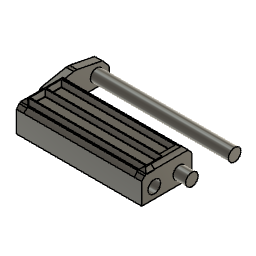
oruga v3 (Autodesk Fusion 360 design; units mm, degrees)
Autodesk Fusion 360 part; units mm, degrees
sketch "Sketch1" plane through (0, 0, 0) normal (0, 0, 1) x (1, 0, 0)
  line L0 (0, 0) -> (50, 0)
  line L1 (50, 0) -> (50, 20)
  line L2 (50, 20) -> (0, 20)
  line L3 (0, 20) -> (0, 0)
  constraint horizontal L0
  constraint vertical L1
  constraint horizontal L2
  constraint vertical L3
  constraint coincident L0.start L3.end
extrude "Extrude1" add sketch "Sketch1" along normal blind 10 contours L0 L1 L2 L3 picked at (16.666667, 13.333333) makes body 1
sketch "Sketch2" plane through (0, 0, 10) normal (0, 0, 1) x (-1, 0, 0)
  line L0 (0, -20) -> (0, 0)
  line L1 (0, 0) -> (-50, 0)
  line L2 (-50, 0) -> (-50, -20)
  line L3 (-50, -20) -> (0, -20)
  line L4 (0, -10) -> (-50, -10)
  line L5 (0, -20) -> (-50, -20)
  line L6 (-50, -20) -> (-50, 0)
  line L7 (-50, 0) -> (0, 0)
  line L8 (0, 0) -> (0, -20)
  line L9 (0, -10) -> (0, -11.5)
  line L10 (0, -10) -> (0, -8.5)
  line L11 (-25, -10) -> (-23.5, -10)
  line L12 (-25, -10) -> (-26.5, -10)
  line L13 (-23.5, -10) -> (-23.5, -20)
  line L14 (-23.5, -10) -> (-23.5, 0)
  line L15 (-26.5, -10) -> (-26.5, 0)
  line L16 (-26.5, -10) -> (-26.5, -20)
  line L17 (0, -20) -> (0, -15)
  line L18 (0, -15) -> (-50, -15)
  line L19 (0, 0) -> (0, -5)
  line L20 (-50, -5) -> (0, -5)
  line L21 (0, -5) -> (0, -2)
  line L22 (0, -2) -> (-1, -2)
  line L23 (-1, -2) -> (-50.000001, -2)
  line L24 (-50, -5) -> (-50.000001, -2)
  line L25 (0, -15) -> (0, -17.5)
  line L26 (0, -15) -> (0, -18)
  line L27 (0, -18) -> (-50, -18)
  line L28 (-50, -18) -> (-50, -15)
  line L29 (0, -10) -> (0, -11.5)
  line L30 (0, -10) -> (0, -8.5)
  line L31 (0, -11.5) -> (-50, -11.5)
  line L32 (0, -8.5) -> (-50, -8.5)
  line L33 (0, -20) -> (-2.713572, -20)
  line L34 (0, -20) -> (0, 0)
  line L35 (0, 0) -> (-2.713572, 0)
  line L36 (0, 0) -> (-2.713572, 0)
  line L37 (-50, -20) -> (-49.000001, -20)
  line L38 (-50, -20) -> (-48.000001, -20)
  line L39 (-50, 0) -> (-48.000001, 0)
  line L40 (0, -20) -> (-3, -20)
  line L41 (-3, -20) -> (-3, 0)
  line L42 (0, 0) -> (-3, 0)
  line L43 (-50, -20) -> (-47.000001, -20)
  line L44 (-47.000001, 0) -> (-47.000001, -20)
  line L45 (-47.000001, 0) -> (-50, 0)
  dimension "d5" = 1.5
  dimension "d6" = 1.5
  dimension "d7" = 3
  dimension "d8" = 3
  dimension "d9" = 1.5
  dimension "d10" = 3
  dimension "d13" = 1.5
  dimension "d22" = 2
  dimension "d23" = 2
  constraint midpoint L0 L4.start
  constraint midpoint L2 L4.end
  constraint horizontal L5
  constraint vertical L6
  constraint horizontal L7
  constraint vertical L8
  constraint coincident L1.end L2.start
  constraint coincident L0.start L3.end
  constraint perpendicular L4 L9
  constraint vertical L10
  constraint midpoint L4 L11.start
  constraint horizontal L11
  constraint horizontal L12
  constraint coincident L5 L13.end
  constraint perpendicular L5 L13
  constraint coincident L1 L14.end
  constraint perpendicular L1 L14
  constraint coincident L7 L15.end
  constraint perpendicular L7 L15
  constraint coincident L5 L16.end
  constraint perpendicular L5 L16
  constraint coincident L8 L17.end
  constraint coincident L6 L18.end
  constraint perpendicular L6 L18
  constraint coincident L0.end L1.start
  constraint coincident L8 L19.end
  constraint coincident L6 L20.start
  constraint perpendicular L0 L20
  constraint perpendicular L20 L21
  constraint perpendicular L8 L22
  constraint perpendicular L8 L23
  constraint perpendicular L23 L24
  constraint midpoint L17 L25.end
  constraint perpendicular L18 L26
  constraint coincident L6 L27.end
  constraint perpendicular L6 L27
  constraint perpendicular L4 L29
  constraint coincident L0 L10.end
  constraint coincident L6 L31.end
  constraint perpendicular L6 L31
  constraint coincident L6 L32.end
  constraint perpendicular L6 L32
  constraint perpendicular L17 L33
  constraint perpendicular L19 L35
  constraint coincident L2.end L3.start
  constraint perpendicular L2 L37
  constraint perpendicular L2 L38
  constraint perpendicular L8 L40
  constraint coincident L1 L41.end
  constraint perpendicular L1 L41
  constraint parallel L3 L43
  constraint perpendicular L5 L44
  measures "d5" distance of L11.start L11.end
  measures "d6" distance of L11.start L12.end
  measures "d7" distance of L19.end L21.end
  measures "d8" distance of L17.end L26.end
  measures "d9" distance of L4.start L9.end
  measures "d10" distance of L0.start L40.end
  measures "d13" distance of L4 L32
  measures "d22" distance of L5 L27
  measures "d23" distance of L7 L23
sketch "Sketch3" plane through (0, 0, 10) normal (0, 0, 1) x (-1, 0, 0)
extrude "Extrude2" add sketch "Sketch2" along normal blind 1.5 contours L0 L3 L5 L8 L17 L27 L33 L34 L40 L41 | L0 L8 L17 L18 L25 L26 L27 L34 L41 | L13 L18 L27 L41 | L0 L8 L18 L31 L34 L41 | L13 L16 L18 L27 | L0 L4 L8 L9 L29 L31 L34 L41 | L16 L18 L27 L44 | L4 L13 L31 L41 | L0 L4 L8 L10 L30 L32 L34 L41 | L4 L11 L12 L13 L16 L31 | L2 L3 L5 L6 L27 L37 L38 L43 L44 | L2 L6 L18 L27 L28 L44 | L4 L14 L32 L41 | L0 L8 L20 L32 L34 L41 | L4 L11 L12 L14 L15 L32 | L4 L16 L31 L44 | L2 L6 L18 L31 L44 | L0 L8 L19 L20 L21 L22 L23 L34 L41 | L4 L15 L32 L44 | L2 L4 L6 L31 L44 | L14 L20 L23 L41 | L0 L1 L7 L8 L19 L22 L23 L34 L35 L36 L41 L42 | L14 L15 L20 L23 | L2 L4 L6 L32 L44 | L15 L20 L23 L44 | L2 L6 L20 L32 L44 | L2 L6 L20 L23 L24 L44 | L1 L2 L6 L7 L23 L39 L44 L45 picked at (-1.904524, -18.666667) picked at (-2, -16.833334) picked at (-9.833333, -17) picked at (-1, -13.833333) picked at (-24.5, -17) picked at (-1, -11) picked at (-40.166667, -17) picked at (-9.833333, -11) picked at (-2, -9) picked at (-25, -11) picked at (-48.333334, -18.666667) picked at (-48, -17) picked at (-9.833333, -9.5) picked at (-1, -7.333333) picked at (-25, -9) picked at (-33.333334, -11) picked at (-48, -13.833333) picked at (-1.333333, -4) picked at (-33.333334, -9.5) picked at (-48, -11) picked at (-9.833333, -4) picked at (-1.237857, -0.666667) picked at (-24.5, -4) picked at (-48, -9.5) picked at (-33.333334, -3) picked at (-48, -7.333333) picked at (-49.000001, -3) picked at (-48.333334, -1.333333) bodies 1
fillet "Fillet2" radius 1.5 tangency weight 0.1 2 edges at (25, 0, 10) (25, 20, 10) on bodies 1
fillet "Fillet3" radius 1.3 tangency weight 0.1 17 edges at (25, 18, 11.5) (25, 15, 11.5) (25, 11.5, 11.5) (25, 8.5, 11.5) (25, 5, 11.5) (25, 2, 11.5) (50, 1, 11.5) (50, 3.5, 11.5) (50, 12.5, 11.5) (47.000001, 6.75, 11.5) (0, 10, 11.5) (3, 13.25, 11.5) (3, 6.75, 11.5) (3, 1, 11.5) (3, 19, 11.5) (47.000001, 1, 11.5) (47.000001, 19, 11.5) on bodies 1
sketch "Sketch4" plane through (47.000001, 0, 0) normal (-1, 0, 0) x (0, -1, 0)
  line L0 (-2, 10.2) -> (0, 10.2)
  line L1 (-2, 10.2) -> (-2, 10)
  line L2 (-2, 10) -> (-1.5, 10)
  spline S0 degree 3 poles (-1.5, 10) (-1.497754, 10) (-1.495245, 9.999497) (-1.485681, 9.996756) (-1.477024, 9.992397) (-1.426244, 9.963783) (-1.35731, 9.908052) (-1.081645, 9.678577) (-0.69535, 9.30536) (-0.253424, 8.83336) (-0.144968, 8.709957) (-0.057473, 8.59808) (-0.032362, 8.564766) (-0.011899, 8.530833) (-0.006983, 8.522077) (-0.001511, 8.508925) (0, 8.50389) (0, 8.5) knots 0 0 0 0 0.00067382 0.00067382 0.0026627 0.0026627 0.01394395 0.01394395 0.0767544 0.0767544 0.10450735 0.10450735 0.11224047 0.11224047 0.11432922 0.11432922 0.1157493 0.1157493 0.1157493 0.1157493
  line L3 (0, 8.5) -> (0, 10.2)
  line L4 (0, 8.5) -> (0, 11.8)
  line L5 (0, 8.5) -> (-1.7, 10.3)
  line L6 (-1.7, 10.3) -> (-3, 11.8)
  line L7 (-3, 11.8) -> (0, 11.8)
  line L8 (-20, 8.5) -> (-20, 11.8)
  line L9 (-20, 11.8) -> (-17, 11.8)
  line L10 (-17, 11.8) -> (-20, 8.5)
  dimension "d30" = 3
  dimension "d31" = 3.3
  dimension "d32" = 3.3
  dimension "d33" = 3
  constraint coincident S0.end L3.start
  constraint perpendicular L4 L7
  constraint vertical L8
  constraint perpendicular L8 L9
  measures "d30" distance of L6.end L4.end
  measures "d31" distance of S0.end L4.end
  measures "d32" distance of L8.start L8.end
  measures "d33" distance of L8.end L9.end
extrude "Extrude3" cut sketch "Sketch4" along normal blind -5 and the other way blind -54 contours L0 L4 L5 L6 L7 | L0 S0 L3 L4 L5 | L8 L9 L10 picked at (-1.566667, 11.3) picked at (-0.597787, 9.720844) picked at (-19, 10.7) bodies 1
sketch "Sketch5" plane through (0, 0, 0) normal (-1, 0, 0) x (0, -1, 0)
  line L0 (-18.454546, 10.2) -> (-20, 8.5)
  line L1 (-20, 8.5) -> (-20, 0)
  line L2 (-20, 0) -> (0, 0)
  line L3 (0, 0) -> (0, 8.5)
  spline S0 degree 3 poles (0, 8.5) (0, 8.502163) (-0.00047, 8.504515) (-0.002526, 8.512081) (-0.005428, 8.518426) (-0.017842, 8.542316) (-0.033486, 8.564986) (-0.108325, 8.667458) (-0.224612, 8.802012) (-0.641443, 9.248729) (-0.975068, 9.575852) (-1.217697, 9.789327) knots 0 0 0 0 0.0006489 0.0006489 0.0023603 0.0023603 0.00768797 0.00768797 0.03123059 0.03123059 0.07250533 0.07250533 0.07250533 0.07250533
  line L4 (-1.217697, 9.789327) -> (-1.605556, 10.2)
  line L5 (-18.454546, 10.2) -> (-1.605556, 10.2)
  line L6 (-20, 4.25) -> (0, 4.25)
  circle A0 centre (-10, 4.25) radius 2.5
  dimension "d38" = 5
  constraint midpoint L1 L6.start
  constraint midpoint L3 L6.end
  constraint midpoint L6 A0.centre
  measures "d38" diameter of A0
fillet "Fillet8" radius 0.2 4 edges at (47.000001, 18.25, 10) (47.000001, 18.741651, 9.824783) (3, 18.766425, 9.803251) (3, 18.25, 10) on bodies 1
fillet "Fillet9" radius 0.2 4 edges at (3, 1.75, 10) (3, 1.363508, 9.912388) (47.000001, 1.352402, 9.903492) (47.000001, 1.75, 10) on bodies 1
sketch "Sketch6" plane through (0, 0, 0) normal (-1, 0, 0) x (0, -1, 0)
  line L0 (-18.454546, 10.2) -> (-20, 8.5)
  line L1 (-20, 8.5) -> (-20, 0)
  line L2 (-20, 0) -> (0, 0)
  line L3 (0, 0) -> (0, 8.5)
  spline S0 degree 3 poles (0, 8.5) (0, 8.502163) (-0.00047, 8.504515) (-0.002526, 8.512081) (-0.005428, 8.518426) (-0.017842, 8.542316) (-0.033486, 8.564986) (-0.108325, 8.667458) (-0.224612, 8.802012) (-0.641443, 9.248729) (-0.975068, 9.575852) (-1.217697, 9.789327) knots 0 0 0 0 0.0006489 0.0006489 0.0023603 0.0023603 0.00768797 0.00768797 0.03123059 0.03123059 0.07250533 0.07250533 0.07250533 0.07250533
  line L4 (-1.217697, 9.789327) -> (-1.605556, 10.2)
  line L5 (-18.454546, 10.2) -> (-1.605556, 10.2)
  line L6 (-20, 4.25) -> (-15, 4.25)
  line L7 (0, 4.25) -> (-5, 4.25)
  circle A0 centre (-15, 4.25) radius 2.5
  circle A1 centre (-5, 4.25) radius 2.5
  dimension "d45" = 5
  dimension "d46" = 5
  dimension "d47" = 5
  dimension "d48" = 5
  constraint midpoint L1 L6.start
  constraint perpendicular L1 L6
  constraint midpoint L3 L7.start
  constraint perpendicular L3 L7
  constraint coincident L6.end A0.centre
  constraint coincident L7.end A1.centre
  measures "d45" distance of L6.start L6.end
  measures "d46" distance of L7.start L7.end
  measures "d47" diameter of A0
  measures "d48" diameter of A1
extrude "Extrude5" cut sketch "Sketch6" against normal blind 60 contours A0 | A1 picked at (-15.407891, 5.629251) picked at (-4.937725, 4.970453) bodies 1
sketch "Sketch7" plane through (0, 0, 0) normal (-1, 0, 0) x (0, -1, 0)
  circle A0 centre (-15, 4.25) radius 2.5
  circle A1 centre (-5, 4.25) radius 2.5
  line L0 (-18.454546, 10.2) -> (-20, 8.5)
  line L1 (-20, 8.5) -> (-20, 0)
  line L2 (-20, 0) -> (0, 0)
  line L3 (0, 0) -> (0, 8.5)
  spline S0 degree 3 poles (0, 8.5) (0, 8.502163) (-0.00047, 8.504515) (-0.002526, 8.512081) (-0.005428, 8.518426) (-0.017842, 8.542316) (-0.033486, 8.564986) (-0.108325, 8.667458) (-0.224612, 8.802012) (-0.641443, 9.248729) (-0.975068, 9.575852) (-1.217697, 9.789327) knots 0 0 0 0 0.0006489 0.0006489 0.0023603 0.0023603 0.00768797 0.00768797 0.03123059 0.03123059 0.07250533 0.07250533 0.07250533 0.07250533
  line L4 (-1.217697, 9.789327) -> (-1.605556, 10.2)
  line L5 (-18.454546, 10.2) -> (-1.605556, 10.2)
  line L6 (-10, 0) -> (-10.030051, 10.2)
  line L7 (-10.030051, 10.2) -> (-37.030051, 10.199999)
  line L8 (-37.030051, 10.199999) -> (-37.03005, -0.000001)
  line L9 (-37.03005, -0.000001) -> (-10, 0)
  line L10 (-15, 4.25) -> (-37.030051, 4.249999)
  line L11 (-37.030051, 4.249999) -> (-32.043051, 4.25)
  circle A2 centre (-32.043051, 4.25) radius 2.5
  circle A3 centre (-15, 4.25) radius 2.5
  dimension "d51" = 27
  dimension "d52" = 10.2
  dimension "d53" = 4.987
  dimension "d54" = 5
  dimension "d55" = 5
  constraint midpoint L2 L6.start
  constraint perpendicular L1 L7
  constraint perpendicular L7 L8
  constraint coincident A0.centre L10.start
  constraint perpendicular L8 L10
  constraint perpendicular L8 L11
  measures "d54" diameter of A2
  measures "d55" diameter of A3
extrude "Extrude6" add sketch "Sketch7" along normal blind 3 separate body contours L0 L1 L2 L5 L6 L7 L9 | L0 L1 L7 L8 L10 L11 A2 | L1 L8 L9 L10 L11 A2 picked at (-14.432591, 9.04767) picked at (-23.21804, 5.912296) picked at (-23.21804, 2.587704) makes body 2
sketch "Sketch8" plane through (0, 0, 0) normal (1, 0, 0) x (0, 1, 0)
  circle A0 centre (32.043051, 4.25) radius 2.5
  circle A1 centre (15, 4.25) radius 2.5
  line L0 (10, 0) -> (37.03005, -0.000001)
  line L1 (37.03005, -0.000001) -> (37.030051, 10.199999)
  line L2 (37.030051, 10.199999) -> (10.030051, 10.2)
  line L3 (10.030051, 10.2) -> (10, 0)
  circle A2 centre (15, 4.25) radius 2.5
  circle A3 centre (32.043051, 4.25) radius 2.5
  constraint concentric A1 A2
  constraint concentric A0 A3
extrude "Extrude7" add sketch "Sketch8" along normal blind 55 and the other way blind 3 contours A0 A3 | A1 A2 picked at (31.800875, 4.917864) picked at (15.519575, 3.458151) bodies 2
sketch "Sketch9" plane through (-3, 0, 0) normal (-1, 0, 0) x (0, -1, 0)
  line L0 (-37.03005, -0.000001) -> (-10, 0)
  line L1 (-10, 0) -> (-10.030051, 10.2)
  line L2 (-10.030051, 10.2) -> (-37.030051, 10.199999)
  line L3 (-37.030051, 10.199999) -> (-37.03005, -0.000001)
  line L4 (-23.530051, 10.2) -> (-37.030051, 7.538863)
  line L5 (-23.530051, 10.2) -> (-10.02218, 7.528289)
extrude "Extrude8" cut sketch "Sketch9" against normal blind 3 contours L2 L3 L4 | L1 L2 L5 picked at (-32.530051, 9.312954) picked at (-14.527427, 9.309429) bodies 2
sketch "Sketch10" plane through (-3, 0, 0) normal (-1, 0, 0) x (0, -1, 0)
  line L0 (-37.030051, 7.538863) -> (-37.03005, -0.000001)
  line L1 (-37.03005, -0.000001) -> (-10, 0)
  line L2 (-10, 0) -> (-10.02218, 7.528289)
  line L3 (-23.515025, 0) -> (-23.515025, -3)
  line L4 (-23.515025, 0) -> (-26.515025, -0.000001)
  line L5 (-23.515025, 0) -> (-20.515025, 0)
  line L6 (-26.515025, -0.000001) -> (-23.515025, -3)
  line L7 (-23.515025, -3) -> (-20.515025, 0)
  line L8 (-23.530051, 10.2) -> (-37.030051, 7.538863)
  line L9 (-10.02218, 7.528289) -> (-23.530051, 10.2)
  dimension "d66" = 3
  dimension "d67" = 3
  dimension "d68" = 3
  constraint perpendicular L1 L3
  constraint perpendicular L3 L4
  constraint perpendicular L3 L5
extrude "Extrude9" add sketch "Sketch10" against normal blind 3 contours L1 L3 L4 L6 | L1 L3 L5 L7 picked at (-24.515025, -1.000001) picked at (-22.515025, -1) bodies 2
fillet "Fillet12" radius 1.5 tangency weight 0.1 2 edges at (-1.5, 37.03005, -0.000001) (-1.5, 10, 0) on bodies 2
fillet "Fillet13" radius 3.5 tangency weight 0.1 3 edges at (-1.5, 37.030051, 7.538863) (-1.5, 23.530051, 10.2) (-1.5, 10.02218, 7.528289) on bodies 2
sketch "Sketch11" plane through (-3, 0, 0) normal (-1, 0, 0) x (0, -1, 0)
  spline S0 degree 3 poles (-12.834612, 8.084558) (-12.829372, 8.083521) (-12.82354, 8.081125) (-12.798939, 8.068962) (-12.774855, 8.051049) (-12.590944, 7.903904) (-12.277347, 7.56) (-11.66749, 6.885871) (-11.024119, 6.106323) (-10.424509, 5.313163) (-10.241409, 5.064595) (-10.095111, 4.833883) (-10.060009, 4.77633) (-10.030911, 4.716748) (-10.023902, 4.701263) (-10.015941, 4.677604) (-10.013754, 4.668487) (-10.013733, 4.661385) knots 0 0 0 0 0.0016023 0.0016023 0.00721984 0.00721984 0.0532903 0.0532903 0.28415744 0.28415744 0.35304229 0.35304229 0.36895789 0.36895789 0.37344792 0.37344792 0.37660074 0.37660074 0.37660074 0.37660074
  line L0 (-12.834612, 8.084558) -> (-22.852092, 10.065907)
  spline S1 degree 3 poles (-24.208096, 10.066342) (-24.202252, 10.067494) (-24.189545, 10.068452) (-24.071513, 10.075408) (-23.740464, 10.079127) (-23.109125, 10.076666) (-22.881806, 10.071784) (-22.852092, 10.065907) knots 0 0 0 0 0.00178691 0.00178691 0.01730205 0.01730205 0.03116062 0.03116062 0.03116062 0.03116062
  line L1 (-24.208096, 10.066342) -> (-34.206949, 8.095356)
  spline S2 degree 3 poles (-37.030051, 4.661436) (-37.030051, 4.666775) (-37.028832, 4.672954) (-37.02169, 4.699357) (-37.008852, 4.726297) (-36.901321, 4.932759) (-36.629291, 5.300396) (-36.083846, 6.031212) (-35.43931, 6.816673) (-34.772245, 7.562386) (-34.561735, 7.791891) (-34.361769, 7.981464) (-34.311616, 8.027374) (-34.258328, 8.067693) (-34.244375, 8.077622) (-34.222538, 8.090057) (-34.213956, 8.093975) (-34.206949, 8.095356) knots 0 0 0 0 0.0016017 0.0016017 0.00719787 0.00719787 0.05272316 0.05272316 0.28051665 0.28051665 0.34873953 0.34873953 0.36449023 0.36449023 0.36892922 0.36892922 0.37204381 0.37204381 0.37204381 0.37204381
  line L2 (-37.030051, 4.661436) -> (-37.03005, 1.499999)
  spline S3 degree 3 poles (-35.53005, -0.000001) (-35.532296, -0.000001) (-35.534805, 0.000503) (-35.544369, 0.003243) (-35.553026, 0.007603) (-35.603806, 0.036216) (-35.672741, 0.091947) (-35.948405, 0.321422) (-36.3347, 0.694639) (-36.776626, 1.166639) (-36.885083, 1.290042) (-36.972578, 1.401919) (-36.997689, 1.435233) (-37.018151, 1.469166) (-37.023068, 1.477922) (-37.028539, 1.491074) (-37.03005, 1.49611) (-37.03005, 1.499999) knots 0 0 0 0 0.00067382 0.00067382 0.0026627 0.0026627 0.01394395 0.01394395 0.0767544 0.0767544 0.10450735 0.10450735 0.11224047 0.11224047 0.11432922 0.11432922 0.1157493 0.1157493 0.1157493 0.1157493
  line L3 (-35.53005, -0.000001) -> (-26.515025, -0.000001)
  line L4 (-26.515025, -0.000001) -> (-23.515025, -3)
  line L5 (-23.515025, -3) -> (-20.515025, 0)
  line L6 (-20.515025, 0) -> (-11.504426, 0)
  spline S4 degree 3 poles (-10.004432, 1.504419) (-10.004426, 1.502174) (-10.004921, 1.499666) (-10.00763, 1.490115) (-10.01195, 1.481479) (-10.040244, 1.430974) (-10.095264, 1.362594) (-10.323685, 1.086977) (-10.69706, 0.69922) (-11.170027, 0.25499) (-11.29382, 0.145854) (-11.406049, 0.05782) (-11.439467, 0.032554) (-11.473503, 0.011969) (-11.482286, 0.007023) (-11.495475, 0.00152) (-11.500525, 0) (-11.504426, 0) knots 0 0 0 0 0.00067364 0.00067364 0.0026574 0.0026574 0.01386035 0.01386035 0.07649553 0.07649553 0.10419068 0.10419068 0.11190428 0.11190428 0.1139867 0.1139867 0.11540198 0.11540198 0.11540198 0.11540198
  line L7 (-10.004432, 1.504419) -> (-10.013733, 4.661385)
  line L8 (-26.515025, -0.000001) -> (-20.515025, 0)
  line L9 (-23.515025, -3) -> (-20.515025, 0)
  line L10 (-26.515025, -0.000001) -> (-23.515025, -3)
extrude "Extrude10" cut sketch "Sketch11" against normal blind 4 contours L4 L5 L8 L9 L10 picked at (-23.515025, -1) bodies 2
